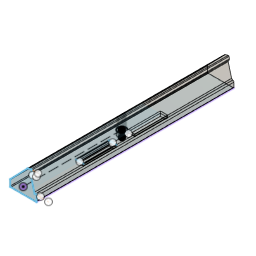
WS2815 LED Holder (Autodesk Fusion 360 design; units mm, degrees)
Autodesk Fusion 360 part; units mm, degrees
note: some values were not read from the file. Chosen so that the rebuilt part matches the saved one: which face or edge a step refers to. Set by a fixed rule: which sketch regions a step uses.
sketch "Profile" plane through (0, 0, 0) normal (0, 1, 0) x (1, 0, 0)
  line L0 (-9.8706, 0) -> (10.1294, 0)
  line L1 (-9.8706, 0) -> (-9.8706, -5)
  line L2 (10.1294, 0) -> (10.1294, -5)
  line L3 (10.1294, -5) -> (8.6805, -4.6118)
  line L4 (10.1294, -5) -> (13.1294, -5) construction
  line L5 (8.6805, -4.6118) -> (5.5747, -16.2029)
  line L6 (8.6805, -4.6118) -> (19.2316, -4.6118) construction
  line L7 (5.5747, -16.2029) -> (7.0236, -16.5911)
  line L8 (5.5747, -16.2029) -> (7.1258, -16.2029) construction
  line L9 (7.0236, -16.5911) -> (6.2471, -19.4889)
  line L10 (7.0236, -16.5911) -> (10.0236, -16.5911) construction
  line L11 (6.2471, -19.4889) -> (3.3493, -18.7124)
  line L12 (6.2471, -19.4889) -> (11.2471, -19.4889) construction
  line L13 (3.3493, -18.7124) -> (-9.8706, -5)
  dimension "d1" = 20
  dimension "d14" = 5
  dimension "d39" = 5
  dimension "d54" = 165
  dimension "d55" = 1.5
  dimension "d56" = 105
  dimension "d57" = 12
  dimension "d58" = 15
  dimension "d59" = 1.5
  dimension "d60" = 105
  dimension "d61" = 3
  dimension "d62" = 165
  dimension "d63" = 3
  constraint horizontal L0
  constraint vertical L1
  constraint vertical L2
  constraint horizontal L4
  constraint horizontal L6
  constraint horizontal L8
  constraint horizontal L10
  constraint horizontal L12
  measures "d1" distance of L0.start L0.end
  measures "d14" distance of L0.start L1.end
  measures "d39" distance of L0.end L2.end
  measures "d54" angle of L3 L4
  measures "d55" distance of L2.end L3.end
  measures "d56" angle of L5 L6
  measures "d57" distance of L3.end L5.end
  measures "d58" angle of L7 L8
  measures "d59" distance of L5.end L7.end
  measures "d60" angle of L9 L10
  measures "d61" distance of L7.end L9.end
  measures "d62" angle of L11 L12
  measures "d63" distance of L9.end L11.end
extrude "Extrude1" add sketch "Profile" along normal blind 150 makes body 1
sketch "Sketch2" plane through (0, 0, 5) normal (0, 0, 1) x (-1, 0, 0)
  line L0 (9.8706, 0) -> (-4.6723, 0)
  line L1 (-4.6723, 0) -> (-4.6723, -100)
  line L2 (-4.6723, -100) -> (9.8706, -100)
  line L3 (9.8706, -100) -> (9.8706, 0)
  line L4 (0, 0) -> (0, -75) construction
  circle A0 centre (0, -75) radius 3
  dimension "d18" = 75
  dimension "d68" = 6
  constraint vertical L4
  constraint coincident L4.start origin
  constraint coincident L4.end A0.centre
  measures "d18" distance of L4.start L4.end
  measures "d68" diameter of A0
hole "Hole1" at (0, 75, 5) direction (0, 0, -1) diameter 3.25 depth 5 tip angle 180 counterbore diameter 6.25 counterbore depth 3.25 bodies 1
sketch "Sketch3" plane through (0, 0, 0) normal (0, 0, -1) x (1, 0, 0)
  circle A0 centre (0, -75) radius 1.625
  line L0 (10.1294, 0) -> (-9.8706, 0)
  line L1 (-9.8706, 0) -> (-9.8706, -150)
  line L2 (-9.8706, -150) -> (10.1294, -150)
  line L3 (0, -75) -> (0, -68) construction
  line L4 (0, -75) -> (0, -80) construction
  line L5 (0, -68) -> (2.75, -68)
  line L6 (2.75, -68) -> (2.75, -43)
  line L7 (2.75, -43) -> (0, -43)
  line L8 (0, -43) -> (0, -68)
  line L9 (0, -68) -> (-2.75, -68)
  line L10 (-2.75, -68) -> (-2.75, -43)
  line L11 (-2.75, -43) -> (0, -43)
  line L12 (10.1294, -150) -> (10.1294, 0)
  dimension "d26" = 2.75
  dimension "d27" = 25
  constraint coincident A0.centre L3.start
  constraint parallel L1 L3
  constraint parallel L3 L4
  constraint horizontal L5
  constraint vertical L6
  constraint horizontal L7
  constraint vertical L8
  constraint symmetric L3.end L8 L5.start
  constraint symmetric L5.end L8 L9.end
  constraint symmetric L6.end L8 L10.end
  constraint symmetric L7.end L8 L11.end
  measures "d26" distance of L3.end L5.end
  measures "d27" distance of L3.end L7.end
extrude "Extrude5" cut sketch "Sketch2" along normal blind 20 contours A0 bodies 1
extrude "Extrude2" add sketch "Sketch3" along normal blind 2.5 separate body contours L5 L6 L7 L8 | L8 L9 L10 L11 makes body 2
mirror "Mirror1" about plane through (0, 68, 0) normal (0, 1, 0) of bodies 2 makes body 3
move_body "Move1" bodies 3 to x (1, 0, 0) y (0, 1, 0) z (0, 0, 1) at (0, 14, 0)
fillet "Fillet3" radius 1 2 faces at (-0.9167, 59.6667, -2.5) (-0.9167, 90.3333, -2.5) on bodies 2 3
combine "Combine1" operation add target body 3 tool bodies 1 2
fillet "Fillet5" radius 1 4 edges at (7.0236, 75, 16.5911) (10.1294, 75, 5) (8.6805, 75, 4.6118) (5.5747, 75, 16.2029) on bodies 3
fillet "Fillet6" radius 0.5 5 edges at (6.2471, 75, 19.4889) (3.3493, 75, 18.7124) (-9.8706, 75, 5) (-9.8706, 75, 0) (10.1294, 75, 0) on bodies 3
equation "d16 = length"
equation "d18 = length / 2"
equation "d39 = d14"
equation "length = 150 mm"
named bodies: "LED Holder", "WS2815 LED Holder"
